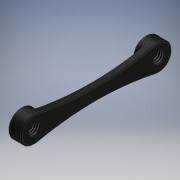
# Autodesk Inventor part: Backplane_CenterNut
Saved by Autodesk Inventor 2018 (Build 220112000, 112)
## iProperties
Created: 2018-10-18
Part Number: Backplane_CenterNut
Material: Aluminum
Document SubType Name: Modeling
Designer: Bradley
Density: 2.7 g/cm^3
Appearance: Anodized - Dark Gray
Author: Bradley
Autodesk Inventor part; units mm, degrees
ref_plane "YZ Plane" through (0, 0, 0) normal (1, 0, 0) x (0, 1, 0)
ref_plane "XZ Plane" through (0, 0, 0) normal (0, 1, 0) x (-1, 0, 0)
ref_plane "XY Plane" through (0, 0, 0) normal (0, 0, 1) x (1, 0, 0)
sketch "Sketch1" plane through (0, 0, 0) normal (1, 0, 0) x (0, 1, 0)
  circle A0 centre (-14, 0) radius 3
  circle A1 centre (14, 0) radius 3
  line L0 (-14, 0) -> (14, 0) construction
  point P0 (0, 0)
  point P1 (0, 0)
  dimension "d0" = 6
  dimension "d1" = 28
  constraints: 2 centre point, 2 end point, 1 coincident, 1 equal radius, 1 horizontal, 1 midpoint
  measures "d0" diameter of A0
  measures "d1" distance of L0.start L0.end
extrude "Extrusion1" add sketch "Sketch1" along normal mid plane 3
sketch "Sketch2" plane through (1.5, 14, 0) normal (1, 0, 0) x (0, 0, -1)
  circle A0 centre (0, -28) radius 3 projected
  circle A1 centre (0, 0) radius 3 projected
  circle A2 centre (0, -28) radius 3 projected
  arc A3 (-2.9319, -27.3644) -> (-2.9319, -0.6356) centre (-64.5833, -14) ccw
  arc A4 (2.9319, -0.6356) -> (2.9319, -27.3644) centre (64.5833, -14) ccw
  circle A5 centre (0, 0) radius 3 projected
  point P0 (0, -14)
  dimension "d4" = 3
  constraints: 8 point on circle, 4 tangent, 2 centre point, 1 equal radius
extrude "Extrusion2" add sketch "Sketch2" against normal blind 1.5 contours A0 A3 A1 A4
sketch "Sketch3" plane through (1.5, 0, 0) normal (1, 0, 0) x (0, 0, -1)
  arc A0 (-2.9319, -13.3644) -> (2.9319, -13.3644) centre (0, -14) ccw projected
  arc A1 (2.9319, 13.3644) -> (2.9319, -13.3644) centre (64.5833, 0) ccw projected
  arc A2 (2.9319, 13.3644) -> (-2.9319, 13.3644) centre (0, 14) ccw projected
  arc A3 (-2.9319, -13.3644) -> (-2.9319, 13.3644) centre (-64.5833, 0) ccw projected
  point P0 (0, 0)
hole "Hole1" at (1.5, 14, 0) at (1.5, -14, 0) direction (-1, 0, 0) diameter 2.459 end through all thread size "M3x0.5" class "6H" standard "ANSI Metric M Profile"
chamfer "Chamfer1" distance 0.25 angle 45 9 edges at (1.5, 0, 1.5) (1.5, -17, 0) (1.5, 0, -1.5) (1.5, 15.8833, -2.3352) (1.5, 15.8833, 2.3352) (-1.5, 11, 0) (-1.5, -17, 0) (0, 0, -1.5) (0, 0, 1.5)
body "Solid1"
